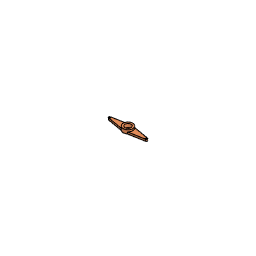
Flight testing can v5 (Autodesk Fusion 360 archive; units mm, degrees)
design "servo_wing"
Autodesk Fusion 360 part; units mm, degrees
sketch "Sketch1" plane through (0, 0, -16) normal (0, 0, -1) x (1, 0, 0)
  arc A0 (-4.6411, 2.2588) -> (-4.984, 2.469) centre (-5.0864, 1.9172) ccw
  arc A1 (-4.984, 2.469) -> (-5.375, 2.375) centre (-5.057, 1.9125) ccw
  arc A2 (-5.375, 2.375) -> (-5.766, 2.469) centre (-5.693, 1.9125) ccw
  arc A3 (-5.766, 2.469) -> (-6.1089, 2.2588) centre (-5.6636, 1.9172) ccw
  arc A4 (-6.1089, 2.2588) -> (-6.5099, 2.2273) centre (-6.2684, 1.7206) ccw
  arc A5 (-6.5099, 2.2273) -> (-6.771, 1.9214) centre (-6.2419, 1.7341) ccw
  arc A6 (-6.771, 1.9214) -> (-7.1426, 1.7676) centre (-6.7564, 1.3604) ccw
  arc A7 (-7.1426, 1.7676) -> (-7.2964, 1.396) centre (-6.7354, 1.3814) ccw
  arc A8 (-7.2964, 1.396) -> (-7.6023, 1.1349) centre (-7.1091, 0.8669) ccw
  arc A9 (-7.6023, 1.1349) -> (-7.6338, 0.7339) centre (-7.0956, 0.8934) ccw
  arc A10 (-7.6338, 0.7339) -> (-7.844, 0.391) centre (-7.2921, 0.2886) ccw
  arc A11 (-7.844, 0.391) -> (-7.75, 0) centre (-7.2875, 0.318) ccw
  arc A12 (-7.75, 0) -> (-7.844, -0.391) centre (-7.2875, -0.318) ccw
  arc A13 (-7.844, -0.391) -> (-7.6338, -0.7339) centre (-7.2921, -0.2886) ccw
  arc A14 (-7.6338, -0.7339) -> (-7.6023, -1.1349) centre (-7.0956, -0.8934) ccw
  arc A15 (-7.6023, -1.1349) -> (-7.2964, -1.396) centre (-7.1091, -0.8669) ccw
  arc A16 (-7.2964, -1.396) -> (-7.1426, -1.7676) centre (-6.7354, -1.3814) ccw
  arc A17 (-7.1426, -1.7676) -> (-6.771, -1.9214) centre (-6.7564, -1.3604) ccw
  arc A18 (-6.771, -1.9214) -> (-6.5099, -2.2273) centre (-6.2419, -1.7341) ccw
  arc A19 (-6.5099, -2.2273) -> (-6.1089, -2.2588) centre (-6.2684, -1.7206) ccw
  arc A20 (-6.1089, -2.2588) -> (-5.766, -2.469) centre (-5.6636, -1.9171) ccw
  arc A21 (-5.766, -2.469) -> (-5.375, -2.375) centre (-5.693, -1.9125) ccw
  arc A22 (-5.375, -2.375) -> (-4.984, -2.469) centre (-5.057, -1.9125) ccw
  arc A23 (-4.984, -2.469) -> (-4.6411, -2.2588) centre (-5.0864, -1.9171) ccw
  arc A24 (-4.6411, -2.2588) -> (-4.2401, -2.2273) centre (-4.4816, -1.7206) ccw
  arc A25 (-4.2401, -2.2273) -> (-3.979, -1.9214) centre (-4.5081, -1.7341) ccw
  arc A26 (-3.979, -1.9214) -> (-3.6074, -1.7676) centre (-3.9936, -1.3604) ccw
  arc A27 (-3.6074, -1.7676) -> (-3.4536, -1.396) centre (-4.0146, -1.3814) ccw
  arc A28 (-3.4536, -1.396) -> (-3.1477, -1.1349) centre (-3.6409, -0.8669) ccw
  arc A29 (-3.1477, -1.1349) -> (-3.1162, -0.7339) centre (-3.6544, -0.8934) ccw
  arc A30 (-3.1162, -0.7339) -> (-2.906, -0.391) centre (-3.4579, -0.2886) ccw
  arc A31 (-2.906, -0.391) -> (-3, 0) centre (-3.4625, -0.318) ccw
  arc A32 (-3, 0) -> (-2.906, 0.391) centre (-3.4625, 0.318) ccw
  arc A33 (-2.906, 0.391) -> (-3.1162, 0.7339) centre (-3.4579, 0.2886) ccw
  arc A34 (-3.1162, 0.7339) -> (-3.1477, 1.1349) centre (-3.6544, 0.8934) ccw
  arc A35 (-3.1477, 1.1349) -> (-3.4536, 1.396) centre (-3.6409, 0.8669) ccw
  arc A36 (-3.4536, 1.396) -> (-3.6074, 1.7676) centre (-4.0146, 1.3814) ccw
  arc A37 (-3.6074, 1.7676) -> (-3.979, 1.9214) centre (-3.9936, 1.3604) ccw
  arc A38 (-3.979, 1.9214) -> (-4.2401, 2.2273) centre (-4.5081, 1.7341) ccw
  arc A39 (-4.2401, 2.2273) -> (-4.6411, 2.2588) centre (-4.4816, 1.7206) ccw
  circle A40 centre (-5.375, 0) radius 1.5
  circle A41 centre (-5.375, 0) radius 1.2295
  circle A42 centre (-5.375, 0) radius 2.5
  circle A43 centre (-5.375, 0) radius 4
  line L0 (-5.375, 0) -> (-5.375, -4) construction
  line L1 (-5.375, 0) -> (-5.375, 4) construction
  line L2 (-5.375, 0) -> (-2.8038, -3.0642) construction
  line L3 (-5.375, 0) -> (-1.375, 0) construction
  line L4 (-5.375, 0) -> (-2.8038, 3.0642) construction
  line L5 (-5.375, 0) -> (-1.375, 0) construction
  line L6 (-5.375, 0) -> (-7.9462, -3.0642) construction
  line L7 (-5.375, 0) -> (-7.9462, 3.0642) construction
  line L8 (-5.375, 0) -> (14.625, 0) construction
  line L9 (-5.375, 0) -> (-25.375, 0) construction
  line L10 (-7.9462, -3.0642) -> (-25.375, 0)
  line L11 (-25.375, 0) -> (-7.9462, 3.0642)
  line L12 (14.625, 0) -> (-2.8038, -3.0642)
  line L13 (-2.8038, 3.0642) -> (14.625, 0)
  line L14 (14.625, 0) -> (9.625, 0) construction
  line L15 (-25.375, 0) -> (-20.375, 0) construction
  circle A44 centre (-20.375, 0) radius 0.5
  circle A45 centre (9.625, 0) radius 0.5
  dimension "d346" = 5
  dimension "d347" = 8
  dimension "d348" = 50
  dimension "d349" = 50
  dimension "d350" = 20
  dimension "d351" = 20
  dimension "d352" = 5
  dimension "d353" = 5
  dimension "d354" = 1
  dimension "d355" = 1
  constraint concentric A40 A42
  constraint concentric A40 A43
  constraint coincident A40.centre A41.centre
  constraint coincident A43 L0.end
  constraint vertical L0
  constraint coincident A43 L1.end
  constraint parallel L0 L1
  constraint horizontal L3
  constraint horizontal L5
  constraint coincident A43 L6.end
  constraint coincident A43 L7.end
  constraint perpendicular L0 L8
  constraint horizontal L9
  constraint parallel L8 L14
  constraint parallel L9 L15
  constraint coincident L15.end A44.centre
  constraint coincident L14.end A45.centre
  measures "d346" diameter of A42
  measures "d347" diameter of A43
  measures "d348" angle of L2 L3
  measures "d349" angle of L4 L5
  measures "d350" distance of A40.centre L8.end
  measures "d351" distance of A40.centre L9.end
  measures "d352" distance of L8.end L14.end
  measures "d353" distance of L9.end L15.end
  measures "d354" diameter of A44
  measures "d355" diameter of A45
extrude "Extrude1" add sketch "Sketch1" against normal blind 3 contours A43
extrude "Extrude2" add sketch "Sketch1" against normal blind 1.5 contours A43 L12 L13 | A43 L10 L11
fillet "Fillet1" radius 0.8 2 edges at (-25.375, 0, -15.25) (14.625, 0, -15.25)

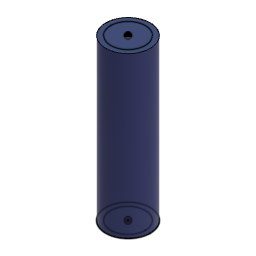
design "Li-ion 18-650"
Autodesk Fusion 360 part; units mm, degrees
sketch "Sketch1" plane through (0, 0, 0) normal (0, 0, 1) x (1, 0, 0)
  circle A0 centre (0, 0) radius 9
  circle A1 centre (0, 0) radius 7
  dimension "d1" = 18
  dimension "d2" = 14
  constraint coincident A0.centre A1.centre
  constraint concentric A0 A1
  measures "d1" diameter of A0
  measures "d2" diameter of A1
extrude "Extrude1" add sketch "Sketch1" along normal blind 65 contours A0 | A1
sketch "Sketch2" plane through (0, 0, 65) normal (0, 0, 1) x (-1, 0, 0)
  circle A0 centre (0, 0) radius 9
  circle A1 centre (0, 0) radius 7
  dimension "d5" = 14
  constraint coincident A0.centre A1.centre
  measures "d5" diameter of A1

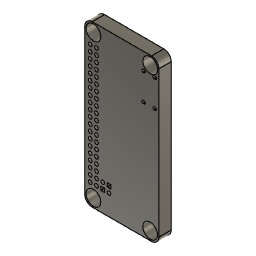
design "RPi shield"
Autodesk Fusion 360 part; units mm, degrees
sketch "Sketch1" plane through (0, 0, 0) normal (0, 1, 0) x (1, 0, 0)
  arc A0 (-14.9458, -100.7564) -> (-11.9458, -103.7564) centre (-11.9458, -100.7564) ccw
  line L0 (-14.9458, -100.7564) -> (-14.9458, -41.7564)
  arc A1 (-11.9458, -38.7564) -> (-14.9458, -41.7564) centre (-11.9458, -41.7564) ccw
  line L1 (-11.9458, -38.7564) -> (12.0542, -38.7564)
  arc A2 (15.0542, -41.7564) -> (12.0542, -38.7564) centre (12.0542, -41.7564) ccw
  line L2 (15.0542, -41.7564) -> (15.0542, -100.7564)
  arc A3 (12.0542, -103.7564) -> (15.0542, -100.7564) centre (12.0542, -100.7564) ccw
  line L3 (12.0542, -103.7564) -> (-11.9458, -103.7564)
  circle A4 centre (11.5542, -100.2564) radius 3
  circle A5 centre (-12.7334, -95.3864) radius 0.75
  circle A6 centre (-12.7334, -92.8464) radius 0.75
  circle A7 centre (-12.7334, -87.7664) radius 0.75
  circle A8 centre (-12.7334, -82.6864) radius 0.75
  circle A9 centre (-12.7334, -77.6064) radius 0.75
  circle A10 centre (-12.7334, -72.5264) radius 0.75
  circle A11 centre (-12.7334, -67.4464) radius 0.75
  circle A12 centre (-12.7334, -62.3664) radius 0.75
  circle A13 centre (-12.7334, -57.2864) radius 0.75
  circle A14 centre (-12.7334, -52.2064) radius 0.75
  circle A15 centre (-12.7334, -47.1264) radius 0.75
  circle A16 centre (-10.1934, -90.3064) radius 0.75
  circle A17 centre (-10.1934, -85.2264) radius 0.75
  circle A18 centre (-10.1934, -80.1464) radius 0.75
  circle A19 centre (-10.1934, -75.0664) radius 0.75
  circle A20 centre (-10.1934, -69.9864) radius 0.75
  circle A21 centre (-10.1934, -64.9064) radius 0.75
  circle A22 centre (-10.1934, -59.8264) radius 0.75
  circle A23 centre (-10.1934, -54.7464) radius 0.75
  circle A24 centre (-10.1934, -49.6664) radius 0.75
  circle A25 centre (-10.1934, -95.3864) radius 0.75
  line L4 (-6.9034, -47.8764) -> (-6.9034, -46.3764)
  line L5 (-6.9034, -46.3764) -> (-8.4034, -46.3764)
  line L6 (-8.4034, -46.3764) -> (-8.4034, -47.8764)
  line L7 (-8.4034, -47.8764) -> (-6.9034, -47.8764)
  circle A26 centre (-11.4458, -42.2564) radius 3
  arc A27 (13.0937, -96.3352) -> (13.0937, -97.3352) centre (13.0937, -96.8352) ccw
  line L8 (13.0937, -97.3352) -> (13.5937, -97.3352)
  arc A28 (13.5937, -97.3352) -> (13.5937, -96.3352) centre (13.5937, -96.8352) ccw
  line L9 (13.5937, -96.3352) -> (13.0937, -96.3352)
  arc A29 (13.0937, -85.4352) -> (13.0937, -86.4352) centre (13.0937, -85.9352) ccw
  line L10 (13.0937, -86.4352) -> (13.5937, -86.4352)
  arc A30 (13.5937, -86.4352) -> (13.5937, -85.4352) centre (13.5937, -85.9352) ccw
  line L11 (13.5937, -85.4352) -> (13.0937, -85.4352)
  arc A31 (8.5937, -85.4352) -> (8.5937, -86.4352) centre (8.5937, -85.9352) ccw
  line L12 (8.5937, -86.4352) -> (9.0937, -86.4352)
  arc A32 (9.0937, -86.4352) -> (9.0937, -85.4352) centre (9.0937, -85.9352) ccw
  line L13 (9.0937, -85.4352) -> (8.5937, -85.4352)
  arc A33 (8.5937, -96.3352) -> (8.5937, -97.3352) centre (8.5937, -96.8352) ccw
  line L14 (8.5937, -97.3352) -> (9.0937, -97.3352)
  arc A34 (9.0937, -97.3352) -> (9.0937, -96.3352) centre (9.0937, -96.8352) ccw
  line L15 (9.0937, -96.3352) -> (8.5937, -96.3352)
  line L16 (-4.3635, -50.3957) -> (-4.3635, -48.8957)
  line L17 (-4.3635, -48.8957) -> (-5.8635, -48.8957)
  line L18 (-5.8635, -48.8957) -> (-5.8635, -50.3957)
  line L19 (-5.8635, -50.3957) -> (-4.3635, -50.3957)
  circle A35 centre (-5.1135, -47.1057) radius 0.75
  circle A36 centre (-10.1934, -47.1264) radius 0.75
  circle A37 centre (-10.1934, -52.2064) radius 0.75
  circle A38 centre (-10.1934, -57.2864) radius 0.75
  circle A39 centre (-10.1934, -62.3664) radius 0.75
  circle A40 centre (-10.1934, -67.4464) radius 0.75
  circle A41 centre (-10.1934, -72.5264) radius 0.75
  circle A42 centre (-10.1934, -77.6064) radius 0.75
  circle A43 centre (-10.1934, -82.6864) radius 0.75
  circle A44 centre (-10.1934, -87.7664) radius 0.75
  circle A45 centre (-10.1934, -92.8464) radius 0.75
  circle A46 centre (-12.7334, -49.6664) radius 0.75
  circle A47 centre (-12.7334, -54.7464) radius 0.75
  circle A48 centre (-12.7334, -59.8264) radius 0.75
  circle A49 centre (-12.7334, -64.9064) radius 0.75
  circle A50 centre (-12.7334, -69.9864) radius 0.75
  circle A51 centre (-12.7334, -75.0664) radius 0.75
  circle A52 centre (-12.7334, -80.1464) radius 0.75
  circle A53 centre (-12.7334, -85.2264) radius 0.75
  circle A54 centre (-12.7334, -90.3064) radius 0.75
  circle A55 centre (-7.6534, -49.6664) radius 0.75
  circle A56 centre (11.5542, -42.2564) radius 3
  circle A57 centre (-11.4458, -100.2564) radius 3
  line L20 (-14.9458, -103.7564) -> (15.0542, -103.7564)
  line L21 (15.0542, -103.7564) -> (15.0542, -38.7564)
  line L22 (15.0542, -38.7564) -> (-14.9458, -38.7564)
  line L23 (-14.9458, -38.7564) -> (-14.9458, -103.7564)
  constraint horizontal L20
  constraint vertical L21
  constraint horizontal L22
  constraint vertical L23
extrude "Extrude1" add sketch "Sketch1" against normal blind 5 contours A0 L0 A1 L1 A2 L2 A3 L3 L20 L21 L22 L23

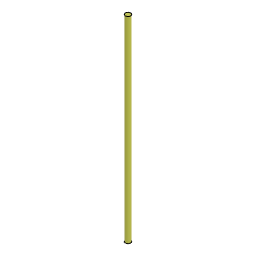
design "threaded_bolt"
Autodesk Fusion 360 part; units mm, degrees
sketch "Sketch1" plane through (0, 0, 0) normal (0, 0, 1) x (1, 0, 0)
  circle A0 centre (0, 0) radius 1.4
  dimension "d190" = 2.8
  constraint coincident A0.centre origin
  measures "d190" diameter of A0
extrude "Extrude1" add sketch "Sketch1" along normal blind 115
move_face "OffsetFaces1" offset -5 4 faces at (0.5063, -0.2629, 0) (0.5063, -0.2629, 0) (0.5063, -0.2629, 0) (0.5063, -0.2629, 0)
thread "Thread1" "ISO Metric profile 3.0 M3x0.5 6g" major diameter 2.927 minor diameter 2.3555 pitch 0.5 angle 60 resizes the face on face at (1.3981, 0.0733, 41.6667)
